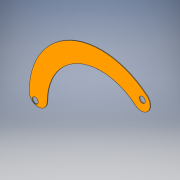
# Autodesk Inventor part: alabes
Saved by Autodesk Inventor 2019 (Build 230136000, 136)
## iProperties
Created: 2020-02-07
Part Number: alabes
Material: Generic
Document SubType Name: Modeling
Designer: Hugo Albarracin
Density: 1 g/cm^3
Appearance: Default
Author: Hugo Albarracin
Autodesk Inventor part; units mm, degrees
ref_plane "YZ Plane" through (0, 0, 0) normal (1, 0, 0) x (0, 1, 0)
ref_plane "XZ Plane" through (0, 0, 0) normal (0, 1, 0) x (-1, 0, 0)
ref_plane "XY Plane" through (0, 0, 0) normal (0, 0, 1) x (1, 0, 0)
sketch "Sketch1" plane through (0, 0, 0) normal (0, 0, 1) x (1, 0, 0)
  arc A0 (77.1345, 91.9253) -> (-120, 0) centre (0, 0) ccw
  arc A1 (57.8509, 68.944) -> (-90, 0) centre (0, 0) ccw
  line L0 (-120, 0) -> (-90, 0) construction
  line L1 (0, 0) -> (77.1345, 91.9253) construction
  line L2 (57.8509, 68.944) -> (77.1345, 91.9253) construction
  arc A2 (-120, 0) -> (-90, 0) centre (-105, 0) ccw
  arc A3 (57.8509, 68.944) -> (77.1345, 91.9253) centre (67.4927, 80.4347) ccw
  dimension "d0" = 240
  dimension "d1" = 30
  dimension "d2" = 130
  constraints: 8 point on circle, 6 end point, 4 centre point, 2 coincident, 2 midpoint, 1 collinear, 1 horizontal, 1 point on line
  measures "d0" diameter of A0
  measures "d1" radial gap between concentric circles of A0 A1
  measures "d2" angle of L1 L0
extrude "Extrusion2" add sketch "Sketch1" along normal blind 1
sketch "Sketch2" plane through (0, 0, 1) normal (0, 0, 1) x (1, 0, 0)
  arc A0 (77.1345, 91.9253) -> (-120, 0) centre (0, 0) ccw projected
  arc A1 (-120, 0) -> (-90, 0) centre (-105, 0) ccw projected
  circle A2 centre (-110, -8) radius 5
  arc A3 (57.8509, 68.944) -> (-90, 0) centre (0, 0) ccw projected
  arc A4 (57.8509, 68.944) -> (77.1345, 91.9253) centre (67.4927, 80.4347) ccw projected
  line L0 (57.8509, 68.944) -> (77.1345, 91.9253) construction
  circle A5 centre (69.4211, 82.7328) radius 5
  line L1 (-120, 0) -> (-90, 0) construction
  line L2 (-120, 0) -> (-120, 14.4317) construction
  line L3 (77.1345, 91.9253) -> (63.1812, 103.6336) construction
  dimension "d10" = 10
  dimension "d12" = 10
  dimension "d20" = 10
  dimension "d21" = 8
  dimension "d22" = 90
  dimension "d23" = 12
  dimension "d24" = 0
  dimension "d25" = 82.7328
  dimension "d26" = 189.4211
  constraints: 8 end point, 2 centre point, 1 horizontal, 1 vertical
  measures "d10" diameter of A2
  measures "d12" diameter of A5
  measures "d20" distance from line of A2.centre L2
  measures "d21" distance from line of A2.centre L1
  measures "d22" angle of L3 L0
  measures "d23" distance from line of A5.centre L3
  measures "d24" distance from line of A5.centre L0
  measures "d25" vertical distance of A5.centre L1.start
  measures "d26" horizontal distance of A5.centre L1.start
extrude "Extrusion3" cut sketch "Sketch2" against normal through all contours A2 | A5
sketch "Sketch3" plane through (0, 0, 1) normal (0, 0, 1) x (1, 0, 0)
  arc A0 (-120, 0) -> (-90, 0) centre (-105, 0) ccw projected
  line L0 (-120, 0) -> (-90, 0) construction
  line L1 (-120, 0) -> (-109.6077, -6)
  line L2 (-109.6077, -6) -> (-91.2523, -6)
  arc A1 (-120, 0) -> (-90, 0) centre (-105, 0) ccw
  point P0 (0, 0)
  dimension "d16" = 30
  dimension "d17" = 6
  constraints: 6 end point, 3 point on circle, 2 horizontal, 1 centre point, 1 coincident
  measures "d16" angle of L0 L1
  measures "d17" distance between parallel lines of L2 L0
extrude "Extrusion4" [suppressed]
equation "\"d0\" = diametro_max"
equation "\"d1\" = ancho_disco"
equation "\"d2\" = angulo_alabe"
equation "\"d10\" = diametro_pin"
equation "\"d12\" = d10"
equation "\"d20\" = desfase_a_pin_inferior"
equation "\"d21\" = desfase_b_pin_inferior"
equation "\"d23\" = desfase_a_pin_superior"
equation "\"angulo_alabe\" = 130deg"
equation "\"ancho_disco\" = 30"
equation "\"diametro_max\" = 240"
equation "\"diametro_tubo\" = 232"
equation "\"desfase_pin_superior\" = 12"
equation "\"desfase_b_pin_inferior\" = 8"
equation "\"desfase_a_pin_inferior\" = 10"
equation "\"desfase_b_pin_superior\" = 0"
equation "\"desfase_a_pin_superior\" = 12"
equation "\"diametro_pin\" = 10"
equation "\"diametro_max_soporte\" = 248"
body "Solid2"
